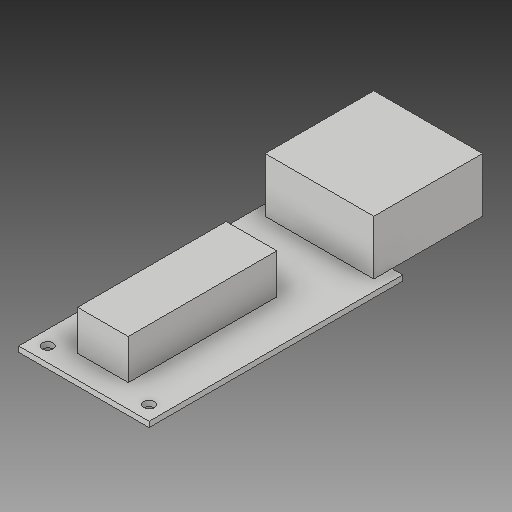
# Autodesk Inventor part: newhub
Saved by Autodesk Inventor 2018 (Build 220112000, 112)
## iProperties
Created: 2017-02-14
Part Number: newhub
Material: Generic
Document SubType Name: Modeling
Designer: steve
Density: 1 g/cm^3
Appearance: Default
Mass: 23.5622 g
Surface Area: 98.68 cm^2
Volume: 23.5622 cm^3
Vendor: Rhoban
Provider: Electronics
Author: steve
Autodesk Inventor part; units mm, degrees
ref_plane "YZ Plane" through (0, 0, 0) normal (1, 0, 0) x (0, 1, 0)
ref_plane "XZ Plane" through (0, 0, 0) normal (0, 1, 0) x (-1, 0, 0)
ref_plane "XY Plane" through (0, 0, 0) normal (0, 0, 1) x (1, 0, 0)
sketch "Sketch1" plane through (0, 0, 0) normal (0, 1, 0) x (-1, 0, 0)
  line L0 (-18, 35) -> (18, 35)
  line L1 (18, 35) -> (18, -35)
  line L2 (18, -35) -> (-18, -35)
  line L3 (-18, -35) -> (-18, 35)
  line L4 (-18, 35) -> (18, -35) construction
  line L5 (18, 35) -> (-18, -35) construction
  point P0 (0, 0)
  dimension "d0" = 70
  dimension "d1" = 36
  constraints: 12 end point, 2 midpoint, 2 parallel, 1 horizontal, 1 perpendicular
  measures "d0" distance of L0.end L1.end
  measures "d1" distance of L0.start L0.end
extrude "Extrusion1" add sketch "Sketch1" along normal blind 1.5
sketch "Sketch2" plane through (0, 1.5, 0) normal (0, 1, 0) x (1, 0, 0)
  line L0 (-48.0959, 5) -> (45.6433, 5) construction
  line L1 (-14, -63.3043) -> (-14, 77.913) construction
  line L2 (14, -60.8696) -> (14, 81.5652) construction
  line L3 (-37.753, -31) -> (38.247, -31) construction
  line L4 (0, 110.5391) -> (0, -92.2783) construction
  circle A0 centre (-14, -31) radius 1.5
  circle A1 centre (14, -31) radius 1.5
  circle A2 centre (-14, 5) radius 1.5
  line L5 (-18, -35) -> (18, -35) projected
  point P0 (0, 0)
  dimension "d4" = 28
  dimension "d5" = 36
  dimension "d6" = 14
  dimension "d7" = 3
  dimension "d8" = 3
  dimension "d9" = 3
  dimension "d10" = 4
  constraints: 8 end point, 6 point on line, 3 centre point, 2 horizontal, 2 vertical
  measures "d4" distance between parallel lines of L2 L1
  measures "d5" distance between parallel lines of L0 L3
  measures "d6" distance between parallel lines of L4 L1
  measures "d7" diameter of A0
  measures "d8" diameter of A2
  measures "d9" diameter of A1
  measures "d10" distance from line of L5 A0.centre
extrude "Extrusion2" cut sketch "Sketch2" against normal through all
sketch "Sketch3" plane through (0, 1.5, 0) normal (0, 1, 0) x (1, 0, 0)
  line L0 (-8.1133, -28.6264) -> (5.8867, -28.6264)
  line L1 (5.8867, -28.6264) -> (5.8867, 12.3736)
  line L2 (5.8867, 12.3736) -> (-8.1133, 12.3736)
  line L3 (-8.1133, 12.3736) -> (-8.1133, -28.6264)
  point P0 (0, 0)
  dimension "d13" = 41
  dimension "d14" = 14
  constraints: 8 end point, 2 parallel, 1 horizontal, 1 perpendicular
  measures "d13" distance of L2.end L0.start
  measures "d14" distance of L0.start L0.end
extrude "Extrusion3" add sketch "Sketch3" along normal blind 11
sketch "Sketch4" plane through (0, 1.5, 0) normal (0, 1, 0) x (1, 0, 0)
  line L0 (-14.9852, 30) -> (15.0148, 30)
  line L1 (15.0148, 30) -> (15.0148, 60)
  line L2 (15.0148, 60) -> (-14.9852, 60)
  line L3 (-14.9852, 60) -> (-14.9852, 30)
  line L4 (18, 35) -> (-18, 35) construction
  point P0 (0, 0)
  dimension "d17" = 30
  dimension "d18" = 30
  dimension "d21" = 5
  constraints: 8 end point, 2 parallel, 1 horizontal, 1 perpendicular
  measures "d17" distance of L1.end L2.end
  measures "d18" distance of L0.end L1.end
  measures "d21" distance between parallel lines of L4 L0
extrude "Extrusion4" add sketch "Sketch4" along normal blind 15
body "Solid1"
